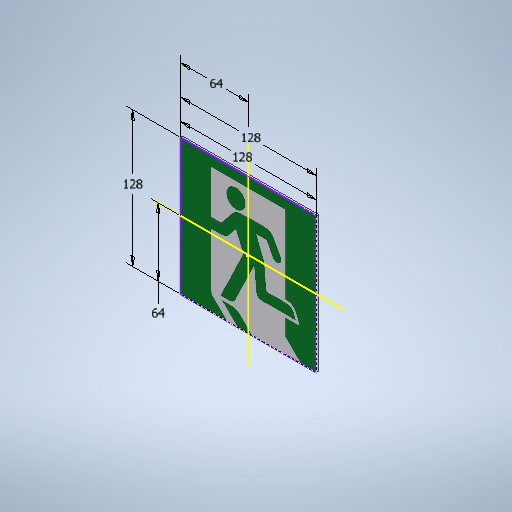
# Autodesk Inventor part: 비장애인
Saved by Autodesk Inventor 2025.1 (Build 291241000, 241)
## iProperties
Created: 2024-10-28
Part Number: 비장애인
Material: 장애인
Document SubType Name: Modeling
Designer: gmsee
Density: 1 g/cm^3
Appearance: 기본값(1)
Author: gmsee
Autodesk Inventor part; units mm, degrees
ref_plane "YZ Plane" through (0, 0, 0) normal (1, 0, 0) x (0, 1, 0)
ref_plane "XZ Plane" through (0, 0, 0) normal (0, 1, 0) x (-1, 0, 0)
ref_plane "XY Plane" through (0, 0, 0) normal (0, 0, 1) x (1, 0, 0)
sketch "스케치1" plane through (0, 0, 0) normal (0, 0, 1) x (1, 0, 0)
  line L0 (0, -89.6) -> (0, 89.6) projected
  line L1 (-89.6, 0) -> (89.6, 0) projected
  line L2 (-64, 64) -> (64, 64)
  line L3 (64, 64) -> (64, -64)
  line L4 (64, -64) -> (-64, -64)
  line L5 (-64, -64) -> (-64, 64)
  line L6 (-64, 64) -> (64, 64) construction
  line L7 (64, 64) -> (64, -64) construction
  line L8 (64, -64) -> (-64, -64) construction
  line L9 (-64, -64) -> (-64, 64) construction
  point P0 (0, 0)
  dimension "d33" = 128
  dimension "d34" = 128
  dimension "d35" = 128
  dimension "d44" = 64
  dimension "d45" = 64
  constraints: 8 end point, 2 parallel, 1 horizontal, 1 perpendicular, 2 other
  measures "d33" distance of L6.start L6.end
  measures "d34" distance of L2.start L2.end
  measures "d35" distance of L4.end L2.start
  measures "d44" distance between parallel lines of L0 L9
  measures "d45" distance between parallel lines of L8 L1
extrude "돌출1" add sketch "스케치1" against normal blind 2
